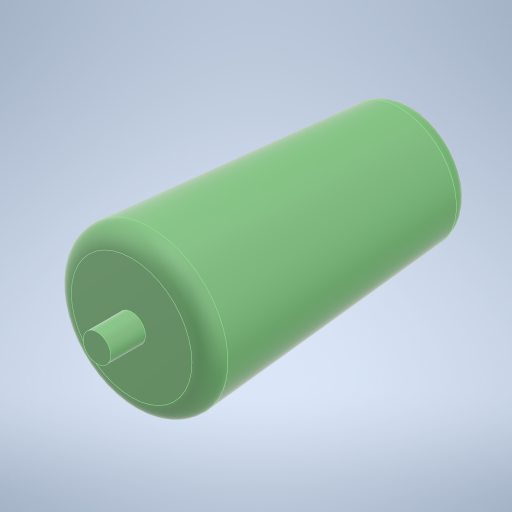
# Autodesk Inventor part: 簡易ピーマン
Saved by Autodesk Inventor 2024 (Build 280153000, 153)
## iProperties
Created: 2024-10-09
Part Number: 簡易ピーマン
Material: 一般
Document SubType Name: Modeling
Designer: hikou
Density: 1 g/cm^3
Appearance: 滑らか - 濃い深緑
Author: hikou
Autodesk Inventor part; units mm, degrees
ref_plane "YZ Plane" through (0, 0, 0) normal (1, 0, 0) x (0, 1, 0)
ref_plane "XZ Plane" through (0, 0, 0) normal (0, 1, 0) x (-1, 0, 0)
sketch "スケッチ1" plane through (0, 0, 0) normal (0, 0, 1) x (1, 0, 0)
  circle A0 centre (0, 0) radius 16.15
  dimension "d0" = 32.3
  constraints: 1 centre point, 1 coincident
  measures "d0" diameter of A0
ref_plane "作業平面2" through (0, 0, 81.7) normal (0, 0, 1) x (1, 0, 0)
sketch "スケッチ3" plane through (0, 0, 81.7) normal (0, 0, 1) x (1, 0, 0)
  circle A0 centre (0, 0) radius 22.8
  dimension "d4" = 45.6
  constraints: 1 centre point, 1 coincident
  measures "d4" diameter of A0
loft "ロフト1" add profiles "スケッチ3", "スケッチ1"
fillet "フィレット1" radius 5 2 edges at (-22.8, 0, 81.7) (-16.15, 0, 0)
sketch "スケッチ4" plane through (0, 0, 81.7) normal (0, 0, 1) x (1, 0, 0)
  circle A0 centre (0, 0) radius 4
  dimension "d10" = 8
  constraints: 1 centre point, 1 coincident
  measures "d10" diameter of A0
extrude "押し出し1" add sketch "スケッチ4" along normal blind 10
